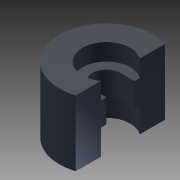
# Autodesk Inventor part: Jig_Bearing_Asm_Holder
Saved by Autodesk Inventor 2011 SP1 (Build 150282100, 282)
## iProperties
Created: 2011-04-25
Part Number: Jig_Bearing_Asm_Holder
Document SubType Name: Modeling
Designer: sungwook
Density: 1 g/cm^3
Author: sungwook
Autodesk Inventor part; units mm, degrees
ref_plane "YZ Plane" through (0, 0, 0) normal (1, 0, 0) x (0, 1, 0)
ref_plane "XZ Plane" through (0, 0, 0) normal (0, 1, 0) x (-1, 0, 0)
ref_plane "XY Plane" through (0, 0, 0) normal (0, 0, 1) x (1, 0, 0)
sketch "Sketch1" plane through (0, 0, 0) normal (0, 0, 1) x (1, 0, 0)
  circle A0 centre (0, 0) radius 5
  dimension "d0" = 10
  constraints: 1 centre point, 1 coincident
  measures "d0" diameter of A0
extrude "Extrusion1" add sketch "Sketch1" along normal blind 5
sketch "Sketch2" plane through (0, 0, 5) normal (0, 0, 1) x (1, 0, 0)
  circle A0 centre (0, 0) radius 5 projected
  arc A1 (0, 1.5) -> (0, -1.5) centre (0, 0) ccw
  line L0 (0, 1.5) -> (4.7697, 1.5)
  line L1 (0, -1.5) -> (4.7697, -1.5)
  arc A2 (4.7697, -1.5) -> (4.7697, 1.5) centre (0, 0) ccw
  dimension "d3" = 3
  constraints: 6 point on circle, 4 end point, 2 centre point, 2 coincident, 2 tangent, 1 horizontal, 1 parallel
  measures "d3" diameter of A1
extrude "Extrusion2" cut sketch "Sketch2" against normal through all contours A0 L1 A1 L0 picked at (1.6667, 0)
sketch "Sketch3" plane through (0, 0, 5) normal (0, 0, 1) x (1, 0, 0)
  arc A0 (0, 1.5) -> (0, -1.5) centre (0, 0) ccw projected
  line L0 (1.5, 5.5246) -> (5.604, 5.5246)
  line L1 (5.604, 5.5246) -> (5.604, -5.9981)
  line L2 (5.604, -5.9981) -> (1.5, -5.9981)
  line L3 (1.5, -5.9981) -> (1.5, 5.5246)
  dimension "d6" = 1.5
  constraints: 8 end point, 2 parallel, 1 horizontal, 1 perpendicular
  measures "d6" distance from line of L3 A0.centre
extrude "Extrusion3" cut sketch "Sketch3" against normal through all
sketch "Sketch4" plane through (0, 0, 0) normal (0, 0, -1) x (-1, 0, 0)
  arc A0 (0, -1.5) -> (0, 1.5) centre (0, 0) ccw projected
  circle A1 centre (0, 0) radius 2.55
  dimension "d9" = 5.1
  constraints: 1 centre point, 1 coincident
  measures "d9" diameter of A1
extrude "Extrusion4" cut sketch "Sketch4" against normal blind 2.7
sketch "Sketch5" plane through (0, 0, 5) normal (0, 0, 1) x (1, 0, 0)
  line L0 (1.5, -4.7697) -> (1.5, -1.5) projected
  line L1 (1.5, -1.5) -> (0, -1.5) projected
  arc A0 (0, 1.5) -> (0, -1.5) centre (0, 0) ccw projected
  line L2 (0, 1.5) -> (1.5, 1.5) projected
  line L3 (1.5, 1.5) -> (1.5, 4.7697) projected
  arc A1 (1.5, 4.7697) -> (1.5, -4.7697) centre (0, 0) ccw projected
extrude "Extrusion5" add sketch "Sketch5" along normal blind 2
sketch "Sketch6" plane through (0, 0, 7) normal (0, 0, 1) x (1, 0, 0)
  arc A0 (1.5, 4.7697) -> (1.5, -4.7697) centre (0, 0) ccw projected
  circle A1 centre (0, 0) radius 2.55
  dimension "d18" = 5.1
  constraints: 1 centre point, 1 coincident
  measures "d18" diameter of A1
extrude "Extrusion6" cut sketch "Sketch6" against normal blind 1.8
body "Solid1"
